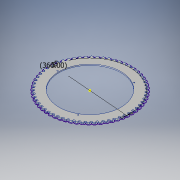
# Autodesk Inventor part: Turret Gear
Saved by Autodesk Inventor 2019.4 (Build 234330000, 330)
## iProperties
Created: 2020-01-22
Part Number: Turret Gear
Material: Aluminum 6061
Document SubType Name: Modeling
Designer: admin
Density: 2.7 g/cm^3
Appearance: Aluminum - Flat
Mass: 617.749 g
Surface Area: 1058.52 cm^2
Volume: 228.796 cm^3
Author: admin
Autodesk Inventor part; units mm, degrees
ref_plane "YZ Plane" through (0, 0, 0) normal (1, 0, 0) x (0, 1, 0)
ref_plane "XZ Plane" through (0, 0, 0) normal (0, 1, 0) x (-1, 0, 0)
ref_plane "XY Plane" through (0, 0, 0) normal (0, 0, 1) x (1, 0, 0)
sketch "Sketch1" plane through (0, 0, 0) normal (0, 1, 0) x (-1, 0, 0)
  circle A0 centre (0, 0) radius 175 construction
  circle A1 centre (0, 0) radius 191.0078 construction
  arc A2 (186.7668, -40.0266) -> (184.3529, -49.7289) centre (185.6551, -44.9015) ccw
  arc A3 (181.4977, -59.309) -> (184.3529, -49.7289) centre (183.0507, -54.5564) ccw
  arc A4 (181.4977, -59.309) -> (178.1449, -68.7266) centre (179.9446, -64.0617) ccw
  arc A5 (174.3039, -77.9558) -> (178.1449, -68.7266) centre (176.3453, -73.3915) ccw
  arc A6 (174.3039, -77.9558) -> (168.0369, -85.1929) centre (172.2626, -82.5201) ccw
  line L0 (0, 0) -> (187.8424, -55.9845)
  line L1 (0, 0) -> (180.9614, -75.3127)
  dimension "d0" = 350
  dimension "d1" = 5
  dimension "d2" = 5
  dimension "d3" = 5
  dimension "d4" = 5
  dimension "d5" = 5
  dimension "d6" = 6
  constraints: 18 point on circle, 7 centre point, 4 end point, 4 equal radius, 2 coincident
  measures "d0" diameter of A0
  measures "d1" radius of A2
  measures "d2" radius of A3
  measures "d3" radius of A4
  measures "d4" radius of A5
  measures "d5" radius of A6
  measures "d6" angle of L0 L1
extrude "Extrusion1" add sketch "Sketch1" along normal blind 5
pattern_circular "Circular Pattern1" count 60 over 360 about axis through (0, 0, 0) along (0, 1, 0) of "Extrusion1"
sketch "Sketch2" plane through (0, 5, 0) normal (0, 1, 0) x (1, 0, 0)
  circle A0 centre (0, 0) radius 148
  dimension "d12" = 296
  constraints: 1 centre point, 1 coincident
  measures "d12" diameter of A0
extrude "Extrusion2" cut sketch "Sketch2" against normal through all
sketch "Sketch3" plane through (0, 5, 0) normal (0, 1, 0) x (1, 0, 0)
  line L0 (-154.73, 0) -> (77.365, 134.0001) construction
  line L1 (77.365, 134.0001) -> (77.365, -134.0001) construction
  line L2 (77.365, -134.0001) -> (-154.73, 0) construction
  circle A0 centre (-154.73, 0) radius 2.75
  circle A1 centre (77.365, 134.0001) radius 2.75
  circle A2 centre (77.365, -134.0001) radius 2.75
  point P0 (0, 0)
  point P1 (0, 0)
  dimension "d15" = 154.73
  dimension "d16" = 5.5
  dimension "d17" = 5.5
  dimension "d18" = 5.5
  constraints: 6 end point, 4 coincident, 3 centre point, 1 vertical, 7 other
  measures "d15" distance of L0.start point (0, 0)
  measures "d16" diameter of A0
  measures "d17" diameter of A1
  measures "d18" diameter of A2
extrude "Extrusion3" cut sketch "Sketch3" against normal through all
sketch "Sketch5" plane through (0, 0, 0) normal (0, 1, 0) x (1, 0, 0)
  arc A0 (-189.8625, 20.2775) -> (-190.6636, 10.3131) centre (-190.3935, 15.3058) ccw construction
  arc A1 (-189.8625, 20.2775) -> (-188.5411, 30.1864) centre (-189.3316, 25.2492) ccw construction
  arc A2 (-186.7029, 40.0125) -> (-188.5411, 30.1864) centre (-187.7506, 35.1235) ccw construction
  line L0 (-187.7506, 35.1235) -> (-192.6654, 36.0429) construction
  arc A3 (-186.7029, 40.0125) -> (-188.5411, 30.1864) centre (-187.7506, 35.1235) ccw construction
  line L1 (-190.3935, 15.3058) -> (-195.3774, 15.7064) construction
  arc A4 (-189.8625, 20.2775) -> (-195.3774, 15.7064) centre (-190.3935, 15.3058) ccw construction
  arc A5 (-189.8625, 20.2775) -> (-188.5411, 30.1864) centre (-189.3316, 25.2492) ccw construction
  arc A6 (-192.6654, 36.0429) -> (-188.5411, 30.1864) centre (-187.7506, 35.1235) ccw construction
  arc A7 (-189.3316, 25.2492) -> (-200.3614, 16.1071) centre (-190.3935, 15.3058) ccw
  arc A8 (-197.5801, 36.9623) -> (-189.3316, 25.2492) centre (-187.7506, 35.1235) ccw
  arc A9 (-190.9336, 5.3204) -> (-200.9474, -4.9246) centre (-190.9504, -4.6796) ccw
  arc A10 (-200.3614, 16.1071) -> (-190.9336, 5.3204) centre (-190.3935, 15.3058) ccw
  arc A11 (-190.4438, -14.6668) -> (-199.3318, -25.9023) centre (-189.4152, -24.6137) ccw
  arc A12 (-200.9474, -4.9246) -> (-190.4438, -14.6668) centre (-190.9504, -4.6796) ccw
  arc A13 (-187.8674, -34.4932) -> (-195.5324, -46.5963) centre (-185.8047, -44.2782) ccw
  arc A14 (-199.3318, -25.9023) -> (-187.8674, -34.4932) centre (-189.4152, -24.6137) ccw
  arc A15 (-183.2328, -53.9418) -> (-189.5906, -66.7797) centre (-180.1586, -63.4575) ccw
  arc A16 (-195.5324, -46.5963) -> (-183.2328, -53.9418) centre (-185.8047, -44.2782) ccw
  arc A17 (-176.5906, -72.7993) -> (-181.5716, -86.2315) centre (-172.5385, -81.9416) ccw
  arc A18 (-189.5906, -66.7797) -> (-176.5906, -72.7993) centre (-180.1586, -63.4575) ccw
  arc A19 (-168.0136, -90.8592) -> (-171.5633, -104.7385) centre (-163.0281, -99.5279) ccw
  arc A20 (-181.5716, -86.2315) -> (-168.0136, -90.8592) centre (-172.5385, -81.9416) ccw
  arc A21 (-157.5958, -107.9237) -> (-159.6753, -122.098) centre (-151.7315, -116.0237) ccw
  arc A22 (-171.5633, -104.7385) -> (-157.5958, -107.9237) centre (-163.0281, -99.5279) ccw
  arc A23 (-145.4514, -123.8057) -> (-146.0378, -138.1198) centre (-138.7725, -131.2484) ccw
  arc A24 (-159.6753, -122.098) -> (-145.4514, -123.8057) centre (-151.7315, -116.0237) ccw
  arc A25 (-131.7134, -138.3313) -> (-130.8004, -152.6282) centre (-124.2931, -145.0351) ccw
  arc A26 (-146.0378, -138.1198) -> (-131.7134, -138.3313) centre (-138.7725, -131.2484) ccw
  arc A27 (-116.5323, -151.3413) -> (-114.1298, -165.4645) centre (-108.452, -157.2327) ccw
  arc A28 (-130.8004, -152.6282) -> (-116.5323, -151.3413) centre (-124.2931, -145.0351) ccw
  arc A29 (-100.0744, -162.6932) -> (-96.2089, -176.4879) centre (-91.4226, -167.7077) ccw
  arc A30 (-114.1298, -165.4645) -> (-100.0744, -162.6932) centre (-108.452, -157.2327) ccw
  arc A31 (-82.5201, -172.2626) -> (-77.2338, -185.5776) centre (-73.3915, -176.3453) ccw
  arc A32 (-96.2089, -176.4879) -> (-82.5201, -172.2626) centre (-91.4226, -167.7077) ccw
  arc A33 (-64.0617, -179.9446) -> (-57.4126, -192.6341) centre (-54.5564, -183.0507) ccw
  arc A34 (-77.2338, -185.5776) -> (-64.0617, -179.9446) centre (-73.3915, -176.3453) ccw
  arc A35 (-44.9015, -185.6551) -> (-36.9623, -197.5801) centre (-35.1235, -187.7506) ccw
  arc A36 (-57.4126, -192.6341) -> (-44.9015, -185.6551) centre (-54.5564, -183.0507) ccw
  arc A37 (-25.2492, -189.3316) -> (-16.1071, -200.3614) centre (-15.3058, -190.3935) ccw
  arc A38 (-36.9623, -197.5801) -> (-25.2492, -189.3316) centre (-35.1235, -187.7506) ccw
  arc A39 (-5.3204, -190.9336) -> (4.9246, -200.9474) centre (4.6796, -190.9504) ccw
  arc A40 (-16.1071, -200.3614) -> (-5.3204, -190.9336) centre (-15.3058, -190.3935) ccw
  arc A41 (14.6668, -190.4438) -> (25.9023, -199.3318) centre (24.6137, -189.4152) ccw
  arc A42 (4.9246, -200.9474) -> (14.6668, -190.4438) centre (4.6796, -190.9504) ccw
  arc A43 (34.4932, -187.8674) -> (46.5963, -195.5324) centre (44.2782, -185.8047) ccw
  arc A44 (25.9023, -199.3318) -> (34.4932, -187.8674) centre (24.6137, -189.4152) ccw
  arc A45 (53.9418, -183.2328) -> (66.7797, -189.5906) centre (63.4575, -180.1586) ccw
  arc A46 (46.5963, -195.5324) -> (53.9418, -183.2328) centre (44.2782, -185.8047) ccw
  arc A47 (72.7993, -176.5906) -> (86.2315, -181.5716) centre (81.9416, -172.5385) ccw
  arc A48 (66.7797, -189.5906) -> (72.7993, -176.5906) centre (63.4575, -180.1586) ccw
  arc A49 (90.8592, -168.0136) -> (104.7385, -171.5633) centre (99.5279, -163.0281) ccw
  arc A50 (86.2315, -181.5716) -> (90.8592, -168.0136) centre (81.9416, -172.5385) ccw
  arc A51 (107.9237, -157.5958) -> (122.098, -159.6753) centre (116.0237, -151.7315) ccw
  arc A52 (104.7385, -171.5633) -> (107.9237, -157.5958) centre (99.5279, -163.0281) ccw
  arc A53 (123.8057, -145.4514) -> (138.1198, -146.0378) centre (131.2484, -138.7725) ccw
  arc A54 (122.098, -159.6753) -> (123.8057, -145.4514) centre (116.0237, -151.7315) ccw
  arc A55 (138.3313, -131.7134) -> (152.6282, -130.8004) centre (145.0351, -124.2931) ccw
  arc A56 (138.1198, -146.0378) -> (138.3313, -131.7134) centre (131.2484, -138.7725) ccw
  arc A57 (151.3413, -116.5323) -> (165.4645, -114.1298) centre (157.2327, -108.452) ccw
  arc A58 (152.6282, -130.8004) -> (151.3413, -116.5323) centre (145.0351, -124.2931) ccw
  arc A59 (162.6932, -100.0744) -> (176.4879, -96.2089) centre (167.7077, -91.4226) ccw
  arc A60 (165.4645, -114.1298) -> (162.6932, -100.0744) centre (157.2327, -108.452) ccw
  arc A61 (172.2626, -82.5201) -> (185.5776, -77.2338) centre (176.3453, -73.3915) ccw
  arc A62 (176.4879, -96.2089) -> (172.2626, -82.5201) centre (167.7077, -91.4226) ccw
  arc A63 (179.9446, -64.0617) -> (192.6341, -57.4126) centre (183.0507, -54.5564) ccw
  arc A64 (185.5776, -77.2338) -> (179.9446, -64.0617) centre (176.3453, -73.3915) ccw
  arc A65 (185.6551, -44.9015) -> (197.5801, -36.9623) centre (187.7506, -35.1235) ccw
  arc A66 (192.6341, -57.4126) -> (185.6551, -44.9015) centre (183.0507, -54.5564) ccw
  arc A67 (189.3316, -25.2492) -> (200.3614, -16.1071) centre (190.3935, -15.3058) ccw
  arc A68 (197.5801, -36.9623) -> (189.3316, -25.2492) centre (187.7506, -35.1235) ccw
  arc A69 (190.9336, -5.3204) -> (200.9474, 4.9246) centre (190.9504, 4.6796) ccw
  arc A70 (200.3614, -16.1071) -> (190.9336, -5.3204) centre (190.3935, -15.3058) ccw
  arc A71 (190.4438, 14.6668) -> (199.3318, 25.9023) centre (189.4152, 24.6137) ccw
  arc A72 (200.9474, 4.9246) -> (190.4438, 14.6668) centre (190.9504, 4.6796) ccw
  arc A73 (187.8674, 34.4932) -> (195.5324, 46.5963) centre (185.8047, 44.2782) ccw
  arc A74 (199.3318, 25.9023) -> (187.8674, 34.4932) centre (189.4152, 24.6137) ccw
  arc A75 (183.2328, 53.9418) -> (189.5906, 66.7797) centre (180.1586, 63.4575) ccw
  arc A76 (195.5324, 46.5963) -> (183.2328, 53.9418) centre (185.8047, 44.2782) ccw
  arc A77 (176.5906, 72.7993) -> (181.5716, 86.2315) centre (172.5385, 81.9416) ccw
  arc A78 (189.5906, 66.7797) -> (176.5906, 72.7993) centre (180.1586, 63.4575) ccw
  arc A79 (168.0136, 90.8592) -> (171.5633, 104.7385) centre (163.0281, 99.5279) ccw
  arc A80 (181.5716, 86.2315) -> (168.0136, 90.8592) centre (172.5385, 81.9416) ccw
  arc A81 (157.5958, 107.9237) -> (159.6753, 122.098) centre (151.7315, 116.0237) ccw
  arc A82 (171.5633, 104.7385) -> (157.5958, 107.9237) centre (163.0281, 99.5279) ccw
  arc A83 (145.4514, 123.8057) -> (146.0378, 138.1198) centre (138.7725, 131.2484) ccw
  arc A84 (159.6753, 122.098) -> (145.4514, 123.8057) centre (151.7315, 116.0237) ccw
  arc A85 (131.7134, 138.3313) -> (130.8004, 152.6282) centre (124.2931, 145.0351) ccw
  arc A86 (146.0378, 138.1198) -> (131.7134, 138.3313) centre (138.7725, 131.2484) ccw
  arc A87 (116.5323, 151.3413) -> (114.1298, 165.4645) centre (108.452, 157.2327) ccw
  arc A88 (130.8004, 152.6282) -> (116.5323, 151.3413) centre (124.2931, 145.0351) ccw
  arc A89 (100.0744, 162.6932) -> (96.2089, 176.4879) centre (91.4226, 167.7077) ccw
  arc A90 (114.1298, 165.4645) -> (100.0744, 162.6932) centre (108.452, 157.2327) ccw
  arc A91 (82.5201, 172.2626) -> (77.2338, 185.5776) centre (73.3915, 176.3453) ccw
  arc A92 (96.2089, 176.4879) -> (82.5201, 172.2626) centre (91.4226, 167.7077) ccw
  arc A93 (64.0617, 179.9446) -> (57.4126, 192.6341) centre (54.5564, 183.0507) ccw
  arc A94 (77.2338, 185.5776) -> (64.0617, 179.9446) centre (73.3915, 176.3453) ccw
  arc A95 (44.9015, 185.6551) -> (36.9623, 197.5801) centre (35.1235, 187.7506) ccw
  arc A96 (57.4126, 192.6341) -> (44.9015, 185.6551) centre (54.5564, 183.0507) ccw
  arc A97 (25.2492, 189.3316) -> (16.1071, 200.3614) centre (15.3058, 190.3935) ccw
  arc A98 (36.9623, 197.5801) -> (25.2492, 189.3316) centre (35.1235, 187.7506) ccw
  arc A99 (5.3204, 190.9336) -> (-4.9246, 200.9474) centre (-4.6796, 190.9504) ccw
  arc A100 (16.1071, 200.3614) -> (5.3204, 190.9336) centre (15.3058, 190.3935) ccw
  arc A101 (-14.6668, 190.4438) -> (-25.9023, 199.3318) centre (-24.6137, 189.4152) ccw
  arc A102 (-4.9246, 200.9474) -> (-14.6668, 190.4438) centre (-4.6796, 190.9504) ccw
  arc A103 (-34.4932, 187.8674) -> (-46.5963, 195.5324) centre (-44.2782, 185.8047) ccw
  arc A104 (-25.9023, 199.3318) -> (-34.4932, 187.8674) centre (-24.6137, 189.4152) ccw
  arc A105 (-53.9418, 183.2328) -> (-66.7797, 189.5906) centre (-63.4575, 180.1586) ccw
  arc A106 (-46.5963, 195.5324) -> (-53.9418, 183.2328) centre (-44.2782, 185.8047) ccw
  arc A107 (-72.7993, 176.5906) -> (-86.2315, 181.5716) centre (-81.9416, 172.5385) ccw
  arc A108 (-66.7797, 189.5906) -> (-72.7993, 176.5906) centre (-63.4575, 180.1586) ccw
  arc A109 (-90.8592, 168.0136) -> (-104.7385, 171.5633) centre (-99.5279, 163.0281) ccw
  arc A110 (-86.2315, 181.5716) -> (-90.8592, 168.0136) centre (-81.9416, 172.5385) ccw
  arc A111 (-107.9237, 157.5958) -> (-122.098, 159.6753) centre (-116.0237, 151.7315) ccw
  arc A112 (-104.7385, 171.5633) -> (-107.9237, 157.5958) centre (-99.5279, 163.0281) ccw
  arc A113 (-123.8057, 145.4514) -> (-138.1198, 146.0378) centre (-131.2484, 138.7725) ccw
  arc A114 (-122.098, 159.6753) -> (-123.8057, 145.4514) centre (-116.0237, 151.7315) ccw
  arc A115 (-138.3313, 131.7134) -> (-152.6282, 130.8004) centre (-145.0351, 124.2931) ccw
  arc A116 (-138.1198, 146.0378) -> (-138.3313, 131.7134) centre (-131.2484, 138.7725) ccw
  arc A117 (-151.3413, 116.5323) -> (-165.4645, 114.1298) centre (-157.2327, 108.452) ccw
  arc A118 (-152.6282, 130.8004) -> (-151.3413, 116.5323) centre (-145.0351, 124.2931) ccw
  arc A119 (-162.6932, 100.0744) -> (-176.4879, 96.2089) centre (-167.7077, 91.4226) ccw
  arc A120 (-165.4645, 114.1298) -> (-162.6932, 100.0744) centre (-157.2327, 108.452) ccw
  arc A121 (-172.2626, 82.5201) -> (-185.5776, 77.2338) centre (-176.3453, 73.3915) ccw
  arc A122 (-176.4879, 96.2089) -> (-172.2626, 82.5201) centre (-167.7077, 91.4226) ccw
  arc A123 (-179.9446, 64.0617) -> (-192.6341, 57.4126) centre (-183.0507, 54.5564) ccw
  arc A124 (-185.5776, 77.2338) -> (-179.9446, 64.0617) centre (-176.3453, 73.3915) ccw
  arc A125 (-185.6551, 44.9015) -> (-197.5801, 36.9623) centre (-187.7506, 35.1235) ccw
  arc A126 (-192.6341, 57.4126) -> (-185.6551, 44.9015) centre (-183.0507, 54.5564) ccw
  point P0 (0, 0)
  point P1 (-189.3316, 25.2492)
  point P2 (-189.3316, 25.2492)
  dimension "d23" = 5
  dimension "d24" = 5
  dimension "d27" = 360
  constraints: 249 point on circle, 123 centre point, 5 coincident, 4 end point, 425 other
  measures "d23" radial gap between concentric circles of A6 A8
  measures "d24" radial gap between concentric circles of A0 A7
body "Solid1"
